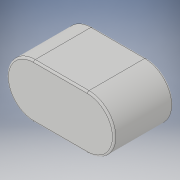
# Autodesk Inventor part: key_sun2
Saved by Autodesk Inventor 2019.4 (Build 234330000, 330)
## iProperties
Created: 2020-01-02
Part Number: key_sun2
Material: 一般
Document SubType Name: Modeling
Designer: Dorian Liu
Density: 1 g/cm^3
Appearance: 預設
Author: Dorian Liu
Autodesk Inventor part; units mm, degrees
ref_plane "YZ Plane" through (0, 0, 0) normal (1, 0, 0) x (0, 1, 0)
ref_plane "XZ Plane" through (0, 0, 0) normal (0, 1, 0) x (-1, 0, 0)
ref_plane "XY Plane" through (0, 0, 0) normal (0, 0, 1) x (1, 0, 0)
sketch "草圖1" plane through (0, 0, 0) normal (0, 0, 1) x (1, 0, 0)
  line L0 (-2.5, -2.5) -> (2.5, -2.5)
  line L1 (2.5, -2.5) -> (2.5, 2.5)
  line L2 (2.5, 2.5) -> (-2.5, 2.5)
  line L3 (-2.5, 2.5) -> (-2.5, -2.5)
  line L4 (-2.5, -2.5) -> (2.5, 2.5) construction
  line L5 (2.5, -2.5) -> (-2.5, 2.5) construction
  arc A0 (2.5, -2.5) -> (2.5, 2.5) centre (2.5, 0) ccw
  arc A1 (-2.5, 2.5) -> (-2.5, -2.5) centre (-2.5, 0) ccw
  point P0 (0, 0)
  dimension "d0" = 5
  dimension "d1" = 5
  constraints: 12 end point, 4 midpoint, 4 point on circle, 2 centre point, 2 parallel, 1 horizontal, 1 perpendicular, 1 point on line
  measures "d0" distance of L2.end L1.end
  measures "d1" distance of L1.end L0.end
extrude "擠出1" add sketch "草圖1" along normal blind 5.5
fillet "圓角1" radius 0.16 8 edges at (-5, 0, 5.5) (0, -2.5, 5.5) (5, 0, 5.5) (0, 2.5, 5.5) (-5, 0, 0) (0, -2.5, 0) (5, 0, 0) (0, 2.5, 0)
